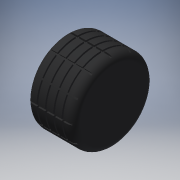
# Autodesk Inventor part: Rubber WheelCJE
Saved by Autodesk Inventor 2018 (Build 220112000, 112)
## iProperties
Created: 2018-02-17
Part Number: Rubber WheelCJE
Material: Rubber
Document SubType Name: Modeling
Designer: textboox5
Density: 0.93 g/cm^3
Appearance: Rubber - Black
Author: textboox5
Autodesk Inventor part; units mm, degrees
ref_plane "YZ Plane" through (0, 0, 0) normal (1, 0, 0) x (0, 1, 0)
sketch "Sketch1" plane through (0, 0, 0) normal (0, 0, 1) x (1, 0, 0)
  line L0 (774.7, 0) -> (1130.3, 0) construction
  line L1 (774.7, 254) -> (774.7, 50.8)
  line L2 (774.7, 50.8) -> (863.6, 50.8)
  line L3 (863.6, 50.8) -> (863.6, 152.4)
  line L4 (863.6, 152.4) -> (1041.4, 152.4)
  line L5 (1041.4, 152.4) -> (1041.4, 0)
  line L6 (1041.4, 0) -> (1130.3, 0)
  line L7 (1130.3, 0) -> (1130.3, 254)
  line L8 (952.5, 0) -> (952.5, 304.8) construction
  line L9 (609.6, 50.8) -> (711.2, 50.8) construction
  line L10 (863.6, 108.0848) -> (863.6, 147.0885) construction
  line L11 (1041.4, 108.0848) -> (1041.4, 147.0885) construction
  arc A0 (825.5, 304.8) -> (774.7, 254) centre (825.5, 254) ccw
  arc A1 (1130.3, 254) -> (1079.5, 304.8) centre (1079.5, 254) ccw
  line L12 (1054.1, 304.8) -> (1054.1, 292.1)
  line L13 (1054.1, 292.1) -> (1041.4, 292.1)
  line L14 (1041.4, 292.1) -> (1041.4, 304.8)
  line L15 (990.6, 304.8) -> (990.6, 292.1)
  line L16 (990.6, 292.1) -> (977.9, 292.1)
  line L17 (977.9, 292.1) -> (977.9, 304.8)
  line L18 (1079.5, 304.8) -> (1054.1, 304.8)
  line L19 (1041.4, 304.8) -> (990.6, 304.8)
  line L20 (850.9, 304.8) -> (850.9, 292.1)
  line L21 (850.9, 292.1) -> (863.6, 292.1)
  line L22 (863.6, 292.1) -> (863.6, 304.8)
  line L23 (914.4, 304.8) -> (914.4, 292.1)
  line L24 (914.4, 292.1) -> (927.1, 292.1)
  line L25 (927.1, 292.1) -> (927.1, 304.8)
  line L26 (977.9, 304.8) -> (927.1, 304.8)
  line L27 (914.4, 304.8) -> (863.6, 304.8)
  line L28 (850.9, 304.8) -> (825.5, 304.8)
  point P0 (0, 0)
  dimension "d0" = 304.8
  dimension "d2" = 355.6
  dimension "d5" = 50.8
  dimension "d7" = 50.8
  dimension "d8" = 12.7
  dimension "d9" = 254
  constraints: 54 end point, 27 perpendicular, 12 tangent, 8 symmetric about line, 7 point on line, 4 collinear, 4 point on circle, 3 equal length, 2 centre point, 2 horizontal, 2 midpoint, 2 vertical, 1 equal radius, 1 parallel, 4 other
  measures "d0" diameter of L4 L0
  measures "d2" distance between parallel lines of L7 L1
  measures "d5" radius of A0
  measures "d7" distance of L14.end L15.start
  measures "d8" distance of L12.end L13.end
  measures "d9" distance between parallel lines of L2 L28
ref_plane "Work Plane1" through (1041.4, 108.0848, 0) normal (1, 0, 0) x (0, 1, 0)
sketch "Sketch2" plane through (1041.4, 108.0848, 0) normal (1, 0, 0) x (0, 1, 0)
  line L0 (-216.1696, -107.4404) -> (-133.4848, -43.9941) projected
  line L1 (-133.4848, -43.9941) -> (-147.0885, -147.3244) projected
  arc A0 (-147.0885, -147.3244) -> (-69.0811, -147.3244) centre (-108.0848, 0) ccw construction
  line L2 (-69.0811, -147.3244) -> (-82.6848, -43.9941) projected
  line L3 (-82.6848, -43.9941) -> (0, -107.4404) projected
  arc A1 (0, -107.4404) -> (39.0037, -39.884) centre (-108.0848, 0) ccw construction
  line L4 (39.0037, -39.884) -> (-57.2848, 0) projected
  line L5 (-57.2848, 0) -> (39.0037, 39.884) projected
  arc A2 (39.0037, 39.884) -> (0, 107.4404) centre (-108.0848, 0) ccw construction
  line L6 (0, 107.4404) -> (-82.6848, 43.9941) projected
  line L7 (-82.6848, 43.9941) -> (-69.0811, 147.3244) projected
  arc A3 (-69.0811, 147.3244) -> (-147.0885, 147.3244) centre (-108.0848, 0) ccw construction
  line L8 (-147.0885, 147.3244) -> (-133.4848, 43.9941) projected
  line L9 (-133.4848, 43.9941) -> (-216.1696, 107.4404) projected
  arc A4 (-216.1696, 107.4404) -> (-255.1733, 39.884) centre (-108.0848, 0) ccw construction
  line L10 (-255.1733, 39.884) -> (-158.8848, 0) projected
  line L11 (-158.8848, 0) -> (-255.1733, -39.884) projected
  arc A5 (-255.1733, -39.884) -> (-216.1696, -107.4404) centre (-108.0848, 0) ccw construction
  arc A6 (39.0037, -39.884) -> (39.0037, 39.884) centre (-108.0848, 0) ccw
  arc A7 (-69.0811, -147.3244) -> (0, -107.4404) centre (-108.0848, 0) ccw
  arc A8 (-216.1696, -107.4404) -> (-147.0885, -147.3244) centre (-108.0848, 0) ccw
  arc A9 (-255.1733, 39.884) -> (-255.1733, -39.884) centre (-108.0848, 0) ccw
  arc A10 (-147.0885, 147.3244) -> (-216.1696, 107.4404) centre (-108.0848, 0) ccw
  arc A11 (0, 107.4404) -> (-69.0811, 147.3244) centre (-108.0848, 0) ccw
  point P0 (-108.0848, 0)
  constraints: 12 point on circle, 6 centre point, 6 coincident
ref_plane "Work Plane2" through (711.2, 25.4, 0) normal (-1, 0, 0) x (0, 0, 1)
ref_plane "Work Plane3" through (812.8, 25.4, 0) normal (-1, 0, 0) x (0, 0, 1)
extrude "Extrusion1" add sketch "Sketch2" against normal up to surface (228.6 mm away)
revolve "Revolution1" add sketch "Sketch1" angle 360 about axis through (774.7, 0, 0) along (1, 0, 0)
sketch "Sketch3" plane through (1130.3, 0, 0) normal (1, 0, 0) x (0, 0, -1)
  line L0 (-6.3208, 304.7345) -> (-6.3208, 292.0345)
  line L1 (-6.3208, 292.0345) -> (6.3792, 292.0345)
  line L2 (6.3792, 292.0345) -> (6.3792, 304.7332)
  circle A0 centre (0, 0) radius 304.8 construction
  circle A1 centre (0, 0) radius 304.8 construction
  line L3 (0.0292, 304.8) -> (0.0292, 292.0345) construction
  arc A2 (6.3792, 304.7332) -> (-6.3208, 304.7345) centre (0, 0) ccw
  line L4 (-157.8412, 260.7474) -> (-151.4912, 249.7489)
  arc A3 (-146.8421, 267.0963) -> (-157.8412, 260.7474) centre (0, 0) ccw
  line L5 (-140.4927, 256.0989) -> (-146.8421, 267.0963)
  line L6 (-151.4912, 249.7489) -> (-140.4927, 256.0989)
  line L7 (-267.0682, 146.8933) -> (-256.0696, 140.5433)
  arc A4 (-260.7171, 157.8912) -> (-267.0682, 146.8933) centre (0, 0) ccw
  line L8 (-249.7196, 151.5418) -> (-260.7171, 157.8912)
  line L9 (-256.0696, 140.5433) -> (-249.7196, 151.5418)
  line L10 (-304.7345, -6.3208) -> (-292.0345, -6.3208)
  arc A5 (-304.7332, 6.3792) -> (-304.7345, -6.3208) centre (0, 0) ccw
  line L11 (-292.0345, 6.3792) -> (-304.7332, 6.3792)
  line L12 (-292.0345, -6.3208) -> (-292.0345, 6.3792)
  line L13 (-260.7474, -157.8412) -> (-249.7489, -151.4912)
  arc A6 (-267.0963, -146.8421) -> (-260.7474, -157.8412) centre (0, 0) ccw
  line L14 (-256.0989, -140.4927) -> (-267.0963, -146.8421)
  line L15 (-249.7489, -151.4912) -> (-256.0989, -140.4927)
  line L16 (-146.8933, -267.0682) -> (-140.5433, -256.0696)
  arc A7 (-157.8912, -260.7171) -> (-146.8933, -267.0682) centre (0, 0) ccw
  line L17 (-151.5418, -249.7196) -> (-157.8912, -260.7171)
  line L18 (-140.5433, -256.0696) -> (-151.5418, -249.7196)
  line L19 (6.3208, -304.7345) -> (6.3208, -292.0345)
  arc A8 (-6.3792, -304.7332) -> (6.3208, -304.7345) centre (0, 0) ccw
  line L20 (-6.3792, -292.0345) -> (-6.3792, -304.7332)
  line L21 (6.3208, -292.0345) -> (-6.3792, -292.0345)
  line L22 (157.8412, -260.7474) -> (151.4912, -249.7489)
  arc A9 (146.8421, -267.0963) -> (157.8412, -260.7474) centre (0, 0) ccw
  line L23 (140.4927, -256.0989) -> (146.8421, -267.0963)
  line L24 (151.4912, -249.7489) -> (140.4927, -256.0989)
  line L25 (267.0682, -146.8933) -> (256.0696, -140.5433)
  arc A10 (260.7171, -157.8912) -> (267.0682, -146.8933) centre (0, 0) ccw
  line L26 (249.7196, -151.5418) -> (260.7171, -157.8912)
  line L27 (256.0696, -140.5433) -> (249.7196, -151.5418)
  line L28 (304.7345, 6.3208) -> (292.0345, 6.3208)
  arc A11 (304.7332, -6.3792) -> (304.7345, 6.3208) centre (0, 0) ccw
  line L29 (292.0345, -6.3792) -> (304.7332, -6.3792)
  line L30 (292.0345, 6.3208) -> (292.0345, -6.3792)
  line L31 (260.7474, 157.8412) -> (249.7489, 151.4912)
  arc A12 (267.0963, 146.8421) -> (260.7474, 157.8412) centre (0, 0) ccw
  line L32 (256.0989, 140.4927) -> (267.0963, 146.8421)
  line L33 (249.7489, 151.4912) -> (256.0989, 140.4927)
  line L34 (146.8933, 267.0682) -> (140.5433, 256.0696)
  arc A13 (157.8912, 260.7171) -> (146.8933, 267.0682) centre (0, 0) ccw
  line L35 (151.5418, 249.7196) -> (157.8912, 260.7171)
  line L36 (140.5433, 256.0696) -> (151.5418, 249.7196)
  point P0 (-145.9919, 252.9239)
  point P1 (-252.8946, 146.0425)
  point P2 (-292.0345, 0.0292)
  point P3 (-252.9239, -145.9919)
  point P4 (-146.0425, -252.8946)
  point P5 (-0.0292, -292.0345)
  point P6 (145.9919, -252.9239)
  point P7 (252.8946, -146.0425)
  point P8 (292.0345, -0.0292)
  point P9 (252.9239, 145.9919)
  point P10 (146.0425, 252.8946)
  dimension "d10" = 12.7
  dimension "d13" = 360
  constraints: 74 end point, 27 point on circle, 12 centre point, 12 midpoint, 4 perpendicular, 1 coincident, 1 vertical, 122 other
  measures "d10" distance of L0.start L0.end
extrude "Extrusion2" cut sketch "Sketch3" against normal through all
body "Solid1"
